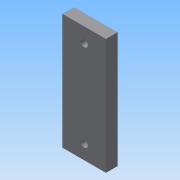
# Autodesk Inventor part: theotherside
Saved by Autodesk Inventor 2015 (Build 190159000, 159)
## iProperties
Created: 2014-09-02
Part Number: theotherside
Material: Generic
Document SubType Name: Modeling
Designer: shohei
Density: 1 g/cm^3
Appearance: Default
Author: shohei
Autodesk Inventor part; units mm, degrees
ref_plane "YZ Plane" through (0, 0, 0) normal (1, 0, 0) x (0, 1, 0)
ref_plane "XZ Plane" through (0, 0, 0) normal (0, 1, 0) x (-1, 0, 0)
ref_plane "XY Plane" through (0, 0, 0) normal (0, 0, 1) x (1, 0, 0)
sketch "Sketch1" plane through (0, 0, 0) normal (0, 1, 0) x (-1, 0, 0)
  line L0 (0, 0) -> (30, 0)
  line L1 (30, 0) -> (30, 80)
  line L2 (30, 80) -> (0, 80)
  line L3 (0, 80) -> (0, 0)
  circle A0 centre (15, 70) radius 2.5
  circle A1 centre (15, 10) radius 2.5
  dimension "d0" = 80
  dimension "d1" = 30
  dimension "d4" = 5
  dimension "d5" = 5
  dimension "d6" = 60
  dimension "d7" = 15
  dimension "d8" = 10
  constraints: 8 end point, 2 centre point, 2 parallel, 1 horizontal, 1 perpendicular
  measures "d0" distance of L0.end L1.end
  measures "d1" distance of L1.end L2.end
  measures "d4" diameter of A0
  measures "d5" diameter of A1
  measures "d6" distance of A0.centre A1.centre
  measures "d7" distance from line of L3 A0.centre
  measures "d8" distance from line of L0 A1.centre
extrude "Extrusion2" add sketch "Sketch1" along normal blind 8
body "Solid2"
